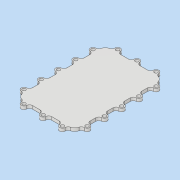
# Autodesk Inventor part: BatteryCaseSide2
Saved by Autodesk Inventor 2017 (Build 210142000, 142)
## iProperties
Created: 2018-02-14
Part Number: BatteryCaseSide2
Material: ABS Plastic
Document SubType Name: Modeling
Designer: Derek Wider
Density: 1.06 g/cm^3
Appearance: Smooth - White
Author: Derek Wider
Autodesk Inventor part; units mm, degrees
ref_plane "YZ Plane" through (0, 0, 0) normal (1, 0, 0) x (0, 1, 0)
ref_plane "XZ Plane" through (0, 0, 0) normal (0, 1, 0) x (-1, 0, 0)
ref_plane "XY Plane" through (0, 0, 0) normal (0, 0, 1) x (1, 0, 0)
sketch "Sketch1" plane through (0, 0, 0) normal (0, 1, 0) x (-1, 0, 0)
  line L0 (4.7625, 0) -> (53.0225, 0)
  line L1 (57.785, -4.7625) -> (57.785, -85.4075)
  line L2 (53.0225, -90.17) -> (4.7625, -90.17)
  line L3 (0, -85.4075) -> (0, -4.7625)
  arc A0 (57.785, -4.7625) -> (53.0225, 0) centre (53.0225, -4.7625) ccw
  arc A1 (4.7625, 0) -> (0, -4.7625) centre (4.7625, -4.7625) ccw
  arc A2 (0, -85.4075) -> (4.7625, -90.17) centre (4.7625, -85.4075) ccw
  arc A3 (53.0225, -90.17) -> (57.785, -85.4075) centre (53.0225, -85.4075) ccw
  line L4 (56.007, -85.4075) -> (56.007, -4.7625)
  arc A4 (56.007, -4.7625) -> (53.0225, -1.778) centre (53.0225, -4.7625) ccw
  line L5 (53.0225, -1.778) -> (4.7625, -1.778)
  arc A5 (4.7625, -1.778) -> (1.778, -4.7625) centre (4.7625, -4.7625) ccw
  line L6 (1.778, -4.7625) -> (1.778, -85.4075)
  arc A6 (1.778, -85.4075) -> (4.7625, -88.392) centre (4.7625, -85.4075) ccw
  line L7 (4.7625, -88.392) -> (53.0225, -88.392)
  arc A7 (53.0225, -88.392) -> (56.007, -85.4075) centre (53.0225, -85.4075) ccw
  line L8 (59.3725, -85.4075) -> (59.3725, -4.7625)
  arc A8 (59.3725, -4.7625) -> (53.0225, 1.5875) centre (53.0225, -4.7625) ccw
  line L9 (53.0225, 1.5875) -> (4.7625, 1.5875)
  arc A9 (4.7625, 1.5875) -> (-1.5875, -4.7625) centre (4.7625, -4.7625) ccw
  line L10 (-1.5875, -4.7625) -> (-1.5875, -85.4075)
  arc A10 (-1.5875, -85.4075) -> (4.7625, -91.7575) centre (4.7625, -85.4075) ccw
  line L11 (4.7625, -91.7575) -> (53.0225, -91.7575)
  arc A11 (53.0225, -91.7575) -> (59.3725, -85.4075) centre (53.0225, -85.4075) ccw
  line L12 (55.245, -4.7625) -> (55.245, -85.4075)
  arc A12 (53.0225, -87.63) -> (55.245, -85.4075) centre (53.0225, -85.4075) ccw
  line L13 (53.0225, -87.63) -> (4.7625, -87.63)
  arc A13 (2.54, -85.4075) -> (4.7625, -87.63) centre (4.7625, -85.4075) ccw
  line L14 (2.54, -85.4075) -> (2.54, -4.7625)
  arc A14 (4.7625, -2.54) -> (2.54, -4.7625) centre (4.7625, -4.7625) ccw
  line L15 (4.7625, -2.54) -> (53.0225, -2.54)
  arc A15 (55.245, -4.7625) -> (53.0225, -2.54) centre (53.0225, -4.7625) ccw
  line L16 (60.1345, -4.7625) -> (60.1345, -85.4075)
  arc A16 (53.0225, -92.5195) -> (60.1345, -85.4075) centre (53.0225, -85.4075) ccw
  line L17 (53.0225, -92.5195) -> (4.7625, -92.5195)
  arc A17 (-2.3495, -85.4075) -> (4.7625, -92.5195) centre (4.7625, -85.4075) ccw
  line L18 (-2.3495, -85.4075) -> (-2.3495, -4.7625)
  arc A18 (4.7625, 2.3495) -> (-2.3495, -4.7625) centre (4.7625, -4.7625) ccw
  line L19 (4.7625, 2.3495) -> (53.0225, 2.3495)
  arc A19 (60.1345, -4.7625) -> (53.0225, 2.3495) centre (53.0225, -4.7625) ccw
  point P0 (0, 0)
  point P1 (57.785, -90.17)
  point P2 (57.785, 0)
  point P3 (0, -90.17)
  dimension "d0" = 90.17
  dimension "d1" = 57.785
  dimension "d2" = 4.7625
  dimension "d3" = 1.778
  dimension "d4" = 1.5875
  dimension "d5" = 0.762
  dimension "d6" = 0.762
  constraints: 40 end point, 40 point on circle, 20 centre point, 10 parallel, 8 point on line, 8 tangent, 5 perpendicular, 3 equal radius, 1 horizontal, 28 other
  measures "d0" distance of point (57.785, 0) point (57.785, -90.17)
  measures "d1" distance of point (57.785, -90.17) point (0, -90.17)
  measures "d2" radius of A0
  measures "d3" distance between parallel lines of L1 L4
  measures "d4" distance between parallel lines of L1 L8
  measures "d5" distance between parallel lines of L4 L12
  measures "d6" distance between parallel lines of L8 L16
extrude "Extrusion1" add sketch "Sketch1" along normal blind 2.159 contours L0 A0 L1 A3 L2 A2 L3 A1 | A7 L7 A6 L6 A5 L5 A4 L4 | A11 L11 A10 L10 A9 L9 A8 L8 | L12 A12 L13 A13 L14 A14 L15 A15
extrude "Extrusion2" add sketch "Sketch1" against normal blind 1.905 contours A7 L7 A6 L6 A5 L5 A4 L4
sketch "Sketch3" plane through (0, 2.159, 0) normal (0, 1, 0) x (1, 0, 0)
  line L0 (1.5875, 4.7625) -> (1.5875, 84.1375) construction
  arc A0 (1.5875, 84.1375) -> (-6.6675, 91.7575) centre (-4.5487, 85.7714) ccw construction
  line L1 (-6.6675, 91.7575) -> (-53.0225, 91.7575) construction
  arc A1 (-53.0225, 91.7575) -> (-59.3725, 84.1375) centre (-53.1511, 85.4088) ccw construction
  line L2 (-59.3725, 84.1375) -> (-59.3725, 4.7625) construction
  arc A2 (-59.3725, 4.7625) -> (-53.0225, -1.5875) centre (-53.0225, 4.7625) ccw construction
  line L3 (-53.0225, -1.5875) -> (-6.6675, -1.5875) construction
  arc A3 (-6.6675, -1.5875) -> (1.5875, 4.7625) centre (-4.7557, 4.4679) ccw construction
  circle A4 centre (-49.2125, 94.6785) radius 1.778
  circle A5 centre (-49.2125, 94.6785) radius 2.921
  circle A6 centre (-28.8925, 94.6785) radius 1.778
  circle A7 centre (-28.8925, 94.6785) radius 2.921
  circle A8 centre (-62.2935, 81.5975) radius 1.778
  circle A9 centre (-62.2935, 81.5975) radius 2.921
  circle A10 centre (-62.2935, 63.3412) radius 1.778
  circle A11 centre (-62.2935, 63.3412) radius 2.921
  line L4 (-28.8925, 94.6785) -> (-28.8925, 104.7777) construction
  circle A12 centre (-62.2935, 45.085) radius 1.778
  circle A13 centre (-62.2935, 45.085) radius 2.921
  circle A14 centre (-62.2935, 26.8287) radius 1.778
  circle A15 centre (-62.2935, 26.8287) radius 2.921
  circle A16 centre (-62.2935, 8.5725) radius 1.778
  circle A17 centre (-62.2935, 8.5725) radius 2.921
  circle A18 centre (-49.2125, -4.5085) radius 1.778
  circle A19 centre (-49.2125, -4.5085) radius 2.921
  circle A20 centre (-28.8925, -4.5085) radius 1.778
  circle A21 centre (-28.8925, -4.5085) radius 2.921
  line L5 (-46.2915, 94.6785) -> (-46.2915, 91.7575)
  line L6 (-6.6675, 91.7575) -> (-53.0225, 91.7575)
  line L7 (-52.1335, 94.6785) -> (-52.1335, 91.7575)
  line L8 (-62.2935, 84.5185) -> (-59.3725, 84.5185)
  line L9 (-62.2935, 78.6765) -> (-59.3725, 78.6765)
  line L10 (-59.3725, 84.5185) -> (-59.3725, 78.6765)
  line L11 (-62.2935, 66.2622) -> (-59.3725, 66.2622)
  line L12 (-62.2935, 60.4202) -> (-59.3725, 60.4202)
  line L13 (-59.3725, 66.2622) -> (-59.3725, 60.4202)
  line L14 (-62.2935, 48.006) -> (-59.3725, 48.006)
  line L15 (-62.2935, 42.164) -> (-59.3725, 42.164)
  line L16 (-59.3725, 48.006) -> (-59.3725, 42.164)
  line L17 (-62.2935, 29.7497) -> (-59.3725, 29.7497)
  line L18 (-62.2935, 23.9077) -> (-59.3725, 23.9077)
  line L19 (-59.3725, 29.7497) -> (-59.3725, 23.9077)
  line L20 (-62.2935, 11.4935) -> (-59.3725, 11.4935)
  line L21 (-62.2935, 5.6515) -> (-59.3725, 5.6515)
  line L22 (-59.3725, 5.6515) -> (-59.3725, 11.4935)
  line L23 (-46.2915, -4.5085) -> (-46.2915, -1.5875)
  line L24 (-52.1335, -4.5085) -> (-52.1335, -1.5875)
  line L25 (-46.2915, -1.5875) -> (-52.1335, -1.5875)
  line L26 (-25.9715, -4.5085) -> (-25.9715, -1.5875)
  line L27 (-31.8135, -4.5085) -> (-31.8135, -1.5875)
  line L28 (-31.8135, -1.5875) -> (-25.9715, -1.5875)
  line L29 (-31.8135, 94.6785) -> (-31.8135, 91.7575)
  line L30 (-25.9715, 94.6785) -> (-25.9715, 91.7575)
  line L31 (-31.8135, 91.7575) -> (-25.9715, 91.7575)
  line L32 (-46.2915, 91.7575) -> (-52.1335, 91.7575)
  line L33 (-51.1175, 91.7575) -> (-4.7625, 91.7575) construction
  circle A22 centre (-8.5725, 94.6785) radius 1.778
  line L34 (-11.4935, 91.7575) -> (-5.6515, 91.7575)
  line L35 (-11.4935, 94.6785) -> (-11.4935, 91.7575)
  circle A23 centre (-8.5725, 94.6785) radius 2.921
  line L36 (-51.1175, 91.7575) -> (-4.7625, 91.7575)
  arc A24 (1.5875, 84.1375) -> (-4.7625, 91.7575) centre (-4.6339, 85.4088) ccw construction
  line L37 (-5.6515, 94.6785) -> (-5.6515, 91.7575)
  line L38 (4.5085, 84.5185) -> (1.5875, 84.5185)
  line L39 (1.5875, 84.5185) -> (1.5875, 78.6765)
  line L40 (4.5085, 78.6765) -> (1.5875, 78.6765)
  circle A25 centre (4.5085, 81.5975) radius 1.778
  circle A26 centre (4.5085, 81.5975) radius 2.921
  circle A27 centre (4.5085, 63.3412) radius 1.778
  line L41 (4.5085, 66.2622) -> (1.5875, 66.2622)
  line L42 (1.5875, 66.2622) -> (1.5875, 60.4202)
  line L43 (4.5085, 60.4202) -> (1.5875, 60.4202)
  circle A28 centre (4.5085, 63.3412) radius 2.921
  line L44 (4.5085, 42.164) -> (1.5875, 42.164)
  circle A29 centre (4.5085, 45.085) radius 1.778
  line L45 (1.5875, 48.006) -> (1.5875, 42.164)
  circle A30 centre (4.5085, 45.085) radius 2.921
  line L46 (4.5085, 48.006) -> (1.5875, 48.006)
  line L47 (4.5085, 23.9077) -> (1.5875, 23.9077)
  circle A31 centre (4.5085, 26.8287) radius 1.778
  line L48 (1.5875, 29.7497) -> (1.5875, 23.9077)
  circle A32 centre (4.5085, 26.8287) radius 2.921
  line L49 (4.5085, 29.7497) -> (1.5875, 29.7497)
  line L50 (1.5875, 84.1375) -> (1.5875, 4.7625) construction
  line L51 (4.5085, 11.4935) -> (1.5875, 11.4935)
  circle A33 centre (4.5085, 8.5725) radius 1.778
  circle A34 centre (4.5085, 8.5725) radius 2.921
  line L52 (1.5875, 5.6515) -> (1.5875, 11.4935)
  line L53 (4.5085, 5.6515) -> (1.5875, 5.6515)
  line L54 (-4.7625, -1.5875) -> (-51.1175, -1.5875) construction
  circle A35 centre (-8.5725, -4.5085) radius 1.778
  circle A36 centre (-8.5725, -4.5085) radius 2.921
  line L55 (-11.4935, -1.5875) -> (-5.6515, -1.5875)
  line L56 (-11.4935, -4.5085) -> (-11.4935, -1.5875)
  line L57 (-5.6515, -4.5085) -> (-5.6515, -1.5875)
  point P0 (0, 0)
  point P1 (0, 0)
  dimension "d11" = 3.556
  dimension "d12" = 5.842
  dimension "d13" = 10.16
  dimension "d14" = 10.16
  dimension "d15" = 18.2563
  dimension "d16" = 10.16
  dimension "d17" = 18.2563
  dimension "d18" = 18.2563
  dimension "d19" = 10.16
  dimension "d26" = 60.96
  dimension "d27" = 93.345
  constraints: 112 end point, 47 symmetric about line, 42 point on circle, 37 centre point, 19 tangent, 16 coincident, 16 equal radius, 16 point on line, 10 perpendicular, 8 horizontal, 5 vertical, 3 collinear, 45 other
  measures "d11" diameter of A4
  measures "d12" diameter of A5
  measures "d14" distance from line of A8.centre L1
  measures "d15" distance of A9.centre A10.centre
  measures "d16" distance from line of L3 A16.centre
  measures "d17" distance of A16.centre A14.centre
  measures "d18" distance of A14.centre A12.centre
  measures "d27" distance between parallel lines of L1 L54
extrude "Extrusion3" add sketch "Sketch3" against normal up to surface (2.159 mm away)
fillet "Fillet1" radius 3.175 32 edges at (-5.6515, 1.0795, -91.7575) (-11.4935, 1.0795, -91.7575) (-25.9715, 1.0795, -91.7575) (-31.8135, 1.0795, -91.7575) (-46.2915, 1.0795, -91.7575) (-52.1335, 1.0795, -91.7575) (-59.3725, 1.0795, -84.5185) (-59.3725, 1.0795, -78.6765) (-59.3725, 1.0795, -66.2622) (-59.3725, 1.0795, -60.4202) (-59.3725, 1.0795, -48.006) (-59.3725, 1.0795, -42.164) (-59.3725, 1.0795, -29.7497) (-59.3725, 1.0795, -23.9077) (-59.3725, 1.0795, -11.4935) (-59.3725, 1.0795, -5.6515) (-52.1335, 1.0795, 1.5875) (-46.2915, 1.0795, 1.5875) (-31.8135, 1.0795, 1.5875) (-25.9715, 1.0795, 1.5875) (-11.4935, 1.0795, 1.5875) (-5.6515, 1.0795, 1.5875) (1.5875, 1.0795, -5.6515) (1.5875, 1.0795, -11.4935) (1.5875, 1.0795, -29.7497) (1.5875, 1.0795, -23.9077) (1.5875, 1.0795, -48.006) (1.5875, 1.0795, -42.164) (1.5875, 1.0795, -60.4202) (1.5875, 1.0795, -66.2622) (1.5875, 1.0795, -78.6765) (1.5875, 1.0795, -84.5185)
sketch "Sketch4" plane through (0, 0, 0) normal (0, -1, 0) x (1, 0, 0)
  arc A0 (-53.0225, -2.54) -> (-55.245, -4.7625) centre (-53.0225, -4.7625) ccw projected
  line L0 (-53.0225, -2.54) -> (-4.7625, -2.54) projected
  arc A1 (-2.54, -4.7625) -> (-4.7625, -2.54) centre (-4.7625, -4.7625) ccw projected
  line L1 (-2.54, -4.7625) -> (-2.54, -85.4075) projected
  arc A2 (-4.7625, -87.63) -> (-2.54, -85.4075) centre (-4.7625, -85.4075) ccw projected
  line L2 (-4.7625, -87.63) -> (-53.0225, -87.63) projected
  arc A3 (-55.245, -85.4075) -> (-53.0225, -87.63) centre (-53.0225, -85.4075) ccw projected
  line L3 (-55.245, -85.4075) -> (-55.245, -4.7625) projected
  line L4 (-56.007, -4.7625) -> (-56.007, -85.4075) projected
  arc A4 (-56.007, -85.4075) -> (-53.0225, -88.392) centre (-53.0225, -85.4075) ccw projected
  line L5 (-53.0225, -88.392) -> (-4.7625, -88.392) projected
  arc A5 (-4.7625, -88.392) -> (-1.778, -85.4075) centre (-4.7625, -85.4075) ccw projected
  line L6 (-1.778, -85.4075) -> (-1.778, -4.7625) projected
  arc A6 (-1.778, -4.7625) -> (-4.7625, -1.778) centre (-4.7625, -4.7625) ccw projected
  line L7 (-4.7625, -1.778) -> (-53.0225, -1.778) projected
  arc A7 (-53.0225, -1.778) -> (-56.007, -4.7625) centre (-53.0225, -4.7625) ccw projected
  line L8 (-58.547, -85.4075) -> (-58.547, -4.7625)
  arc A8 (-53.0225, 0.762) -> (-58.547, -4.7625) centre (-53.0225, -4.7625) ccw
  line L9 (-53.0225, 0.762) -> (-4.7625, 0.762)
  arc A9 (0.762, -4.7625) -> (-4.7625, 0.762) centre (-4.7625, -4.7625) ccw
  line L10 (0.762, -4.7625) -> (0.762, -85.4075)
  arc A10 (-4.7625, -90.932) -> (0.762, -85.4075) centre (-4.7625, -85.4075) ccw
  line L11 (-4.7625, -90.932) -> (-53.0225, -90.932)
  arc A11 (-58.547, -85.4075) -> (-53.0225, -90.932) centre (-53.0225, -85.4075) ccw
  circle A12 centre (-28.8925, 4.5085) radius 1.778 projected
  circle A13 centre (-8.5725, 4.5085) radius 1.778 projected
  circle A14 centre (4.5085, -8.5725) radius 1.778 projected
  circle A15 centre (4.5085, -45.085) radius 1.778 projected
  circle A16 centre (4.5085, -81.5975) radius 1.778 projected
  circle A17 centre (-62.2935, -8.5725) radius 1.778 projected
  circle A18 centre (-62.2935, -81.5975) radius 1.778 projected
  circle A19 centre (-62.2935, -45.085) radius 1.778 projected
  circle A20 centre (-49.2125, -94.6785) radius 1.778 projected
  circle A21 centre (-28.8925, -94.6785) radius 1.778 projected
  circle A22 centre (-8.5725, -94.6785) radius 1.778 projected
  circle A23 centre (-62.2935, -26.8287) radius 1.778 projected
  circle A24 centre (-62.2935, -63.3412) radius 1.778 projected
  circle A25 centre (-49.2125, 4.5085) radius 1.778 projected
  circle A26 centre (4.5085, -63.3412) radius 1.778 projected
  circle A27 centre (4.5085, -26.8287) radius 1.778 projected
  arc A28 (-59.1869, -86.9315) -> (-54.5465, -91.5719) centre (-53.0225, -85.4075) ccw projected
  arc A29 (-52.1335, -94.6541) -> (-54.5465, -91.5719) centre (-55.3085, -94.6541) ccw projected
  arc A30 (-52.1335, -94.6785) -> (-46.294, -94.8002) centre (-49.2125, -94.6785) ccw projected
  arc A31 (-43.1218, -91.7575) -> (-46.294, -94.8002) centre (-43.1218, -94.9325) ccw projected
  line L12 (-34.9832, -91.7575) -> (-43.1218, -91.7575) projected
  arc A32 (-31.811, -94.8002) -> (-34.9832, -91.7575) centre (-34.9832, -94.9325) ccw projected
  arc A33 (-31.811, -94.8002) -> (-25.974, -94.8002) centre (-28.8925, -94.6785) ccw projected
  arc A34 (-22.8018, -91.7575) -> (-25.974, -94.8002) centre (-22.8018, -94.9325) ccw projected
  line L13 (-14.6632, -91.7575) -> (-22.8018, -91.7575) projected
  arc A35 (-11.491, -94.8002) -> (-14.6632, -91.7575) centre (-14.6632, -94.9325) ccw projected
  arc A36 (-11.491, -94.8002) -> (-5.6515, -94.6785) centre (-8.5725, -94.6785) ccw projected
  arc A37 (-3.2385, -91.5719) -> (-5.6515, -94.6541) centre (-2.4765, -94.6541) ccw projected
  arc A38 (-3.2385, -91.5719) -> (1.4019, -86.9315) centre (-4.7625, -85.4075) ccw projected
  arc A39 (4.4841, -84.5185) -> (1.4019, -86.9315) centre (4.4841, -87.6935) ccw projected
  arc A40 (4.5085, -84.5185) -> (4.6302, -78.679) centre (4.5085, -81.5975) ccw projected
  arc A41 (1.5875, -75.5068) -> (4.6302, -78.679) centre (4.7625, -75.5068) ccw projected
  line L14 (1.5875, -69.432) -> (1.5875, -75.5068) projected
  arc A42 (4.6302, -66.2597) -> (1.5875, -69.432) centre (4.7625, -69.432) ccw projected
  arc A43 (4.6302, -66.2597) -> (4.6302, -60.4228) centre (4.5085, -63.3412) ccw projected
  arc A44 (1.5875, -57.2505) -> (4.6302, -60.4228) centre (4.7625, -57.2505) ccw projected
  line L15 (1.5875, -51.1757) -> (1.5875, -57.2505) projected
  arc A45 (4.6302, -48.0035) -> (1.5875, -51.1757) centre (4.7625, -51.1757) ccw projected
  arc A46 (4.6302, -48.0035) -> (4.6302, -42.1665) centre (4.5085, -45.085) ccw projected
  arc A47 (1.5875, -38.9943) -> (4.6302, -42.1665) centre (4.7625, -38.9943) ccw projected
  line L16 (1.5875, -32.9195) -> (1.5875, -38.9943) projected
  arc A48 (4.6302, -29.7472) -> (1.5875, -32.9195) centre (4.7625, -32.9195) ccw projected
  arc A49 (4.6302, -29.7472) -> (4.6302, -23.9103) centre (4.5085, -26.8287) ccw projected
  arc A50 (1.5875, -20.738) -> (4.6302, -23.9103) centre (4.7625, -20.738) ccw projected
  line L17 (1.5875, -14.6632) -> (1.5875, -20.738) projected
  arc A51 (4.6302, -11.491) -> (1.5875, -14.6632) centre (4.7625, -14.6632) ccw projected
  arc A52 (4.6302, -11.491) -> (4.5085, -5.6515) centre (4.5085, -8.5725) ccw projected
  line L18 (4.4841, -5.6515) -> (4.5085, -5.6515) projected
  arc A53 (1.4019, -3.2385) -> (4.4841, -5.6515) centre (4.4841, -2.4765) ccw projected
  arc A54 (1.4019, -3.2385) -> (-3.2385, 1.4019) centre (-4.7625, -4.7625) ccw projected
  arc A55 (-5.6515, 4.4841) -> (-3.2385, 1.4019) centre (-2.4765, 4.4841) ccw projected
  line L19 (-5.6515, 4.5085) -> (-5.6515, 4.4841) projected
  arc A56 (-5.6515, 4.5085) -> (-11.491, 4.6302) centre (-8.5725, 4.5085) ccw projected
  arc A57 (-14.6632, 1.5875) -> (-11.491, 4.6302) centre (-14.6632, 4.7625) ccw projected
  line L20 (-22.8018, 1.5875) -> (-14.6632, 1.5875) projected
  arc A58 (-25.974, 4.6302) -> (-22.8018, 1.5875) centre (-22.8018, 4.7625) ccw projected
  arc A59 (-25.974, 4.6302) -> (-31.811, 4.6302) centre (-28.8925, 4.5085) ccw projected
  arc A60 (-34.9832, 1.5875) -> (-31.811, 4.6302) centre (-34.9832, 4.7625) ccw projected
  line L21 (-43.1218, 1.5875) -> (-34.9832, 1.5875) projected
  arc A61 (-46.294, 4.6302) -> (-43.1218, 1.5875) centre (-43.1218, 4.7625) ccw projected
  arc A62 (-46.294, 4.6302) -> (-52.1335, 4.5085) centre (-49.2125, 4.5085) ccw projected
  arc A63 (-54.5465, 1.4019) -> (-52.1335, 4.4841) centre (-55.3085, 4.4841) ccw projected
  arc A64 (-54.5465, 1.4019) -> (-59.1869, -3.2385) centre (-53.0225, -4.7625) ccw projected
  arc A65 (-62.2691, -5.6515) -> (-59.1869, -3.2385) centre (-62.2691, -2.4765) ccw projected
  arc A66 (-62.2935, -5.6515) -> (-62.4152, -11.491) centre (-62.2935, -8.5725) ccw projected
  arc A67 (-59.3725, -14.6632) -> (-62.4152, -11.491) centre (-62.5475, -14.6632) ccw projected
  line L22 (-59.3725, -20.738) -> (-59.3725, -14.6632) projected
  arc A68 (-62.4152, -23.9103) -> (-59.3725, -20.738) centre (-62.5475, -20.738) ccw projected
  arc A69 (-62.4152, -23.9103) -> (-62.4152, -29.7472) centre (-62.2935, -26.8287) ccw projected
  arc A70 (-59.3725, -32.9195) -> (-62.4152, -29.7472) centre (-62.5475, -32.9195) ccw projected
  line L23 (-59.3725, -38.9943) -> (-59.3725, -32.9195) projected
  arc A71 (-62.4152, -42.1665) -> (-59.3725, -38.9943) centre (-62.5475, -38.9943) ccw projected
  arc A72 (-62.4152, -42.1665) -> (-62.4152, -48.0035) centre (-62.2935, -45.085) ccw projected
  arc A73 (-59.3725, -51.1757) -> (-62.4152, -48.0035) centre (-62.5475, -51.1757) ccw projected
  line L24 (-59.3725, -57.2505) -> (-59.3725, -51.1757) projected
  arc A74 (-62.4152, -60.4228) -> (-59.3725, -57.2505) centre (-62.5475, -57.2505) ccw projected
  arc A75 (-62.4152, -60.4228) -> (-62.4152, -66.2597) centre (-62.2935, -63.3412) ccw projected
  arc A76 (-59.3725, -69.432) -> (-62.4152, -66.2597) centre (-62.5475, -69.432) ccw projected
  line L25 (-59.3725, -75.5068) -> (-59.3725, -69.432) projected
  arc A77 (-62.4152, -78.679) -> (-59.3725, -75.5068) centre (-62.5475, -75.5068) ccw projected
  arc A78 (-62.4152, -78.679) -> (-62.2935, -84.5185) centre (-62.2935, -81.5975) ccw projected
  arc A79 (-59.1869, -86.9315) -> (-62.2691, -84.5185) centre (-62.2691, -87.6935) ccw projected
  arc A80 (-53.0225, -1.778) -> (-56.007, -4.7625) centre (-53.0225, -4.7625) ccw projected
  line L26 (-53.0225, -1.778) -> (-4.7625, -1.778) projected
  arc A81 (-1.778, -4.7625) -> (-4.7625, -1.778) centre (-4.7625, -4.7625) ccw projected
  line L27 (-1.778, -4.7625) -> (-1.778, -85.4075) projected
  arc A82 (-4.7625, -88.392) -> (-1.778, -85.4075) centre (-4.7625, -85.4075) ccw projected
  line L28 (-4.7625, -88.392) -> (-53.0225, -88.392) projected
  arc A83 (-56.007, -85.4075) -> (-53.0225, -88.392) centre (-53.0225, -85.4075) ccw projected
  line L29 (-56.007, -85.4075) -> (-56.007, -4.7625) projected
  line L30 (-52.1335, 4.4841) -> (-52.1335, 4.5085) projected
  line L31 (-62.2935, -5.6515) -> (-62.2691, -5.6515) projected
  line L32 (-52.1335, -94.6785) -> (-52.1335, -94.6541) projected
  line L33 (-5.6515, -94.6541) -> (-5.6515, -94.6785) projected
  line L34 (4.5085, -84.5185) -> (4.4841, -84.5185) projected
  line L35 (-62.2691, -84.5185) -> (-62.2935, -84.5185) projected
  point P0 (0, 0)
  dimension "d23" = 2.54
  constraints: 8 end point, 8 point on circle, 4 centre point, 7 other
  measures "d23" distance between parallel lines of L4 L8
extrude "Extrusion4" add sketch "Sketch4" along normal blind 1.143 contours A79 L35 A78 A77 L25 A76 A75 A74 L24 A73 A72 A71 L23 A70 A69 A68 L22 A67 A66 L31 A65 A64 A63 L30 A62 A61 L21 A60 A59 A58 L20 A57 A56 L19 A55 A54 A53 L18 A52 A51 L17 A50 A49 A48 L16 A47 A46 A45 L15 A44 A43 A42 L14 A41 A40 L34 A39 A38 A37 L33 A36 A35 L13 A34 A33 A32 L12 A31 A30 L32 A29 A28
equation "\"d15\" = d18"
equation "\"d18\" = d17"
equation "\"d19\" = d13"
body "Solid1"
